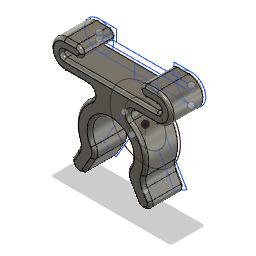
rPi Cable Clip IKEA JANSJO (Autodesk Fusion 360 design; units mm, degrees)
Autodesk Fusion 360 part; units mm, degrees
note: some values were not read from the file. Chosen so that the rebuilt part matches the saved one: a direction. Set by a fixed rule: which sketch regions a step uses.
sketch "Sketch1" plane through (0, 0, 0) normal (0, 0, 1) x (1, 0, 0) in component "Clip"
  circle A0 centre (0, 0) radius 3.6
  circle A1 centre (0, 0) radius 6.1
  line L0 (-1.8246, 8.2256) -> (2.1754, 8.2256)
  line L1 (2.1754, 8.2256) -> (2.1754, 5.6989)
  line L2 (2.1754, 5.6989) -> (-1.8246, 5.6989)
  line L3 (-1.8246, 5.6989) -> (-1.8246, 8.2256)
  line L4 (-8, 9.8345) -> (8, 9.8345)
  line L5 (8, 9.8345) -> (8, 8.8345)
  line L6 (8, 8.8345) -> (-8, 8.8345)
  line L7 (-8, 8.8345) -> (-8, 9.8345)
  circle A2 centre (-8, 9.3345) radius 0.5
  circle A3 centre (8, 9.3345) radius 0.5
  circle A4 centre (-8, 9.3345) radius 2.5
  circle A5 centre (8, 9.3345) radius 2.5
  line L8 (-8, 11.8345) -> (-5, 11.8345)
  line L9 (-5, 11.8345) -> (-5, 9.8345)
  line L10 (-5, 9.8345) -> (-8, 9.8345)
  line L11 (8, 11.8345) -> (5, 11.8345)
  line L12 (5, 11.8345) -> (5, 9.8345)
  line L13 (5, 9.8345) -> (8, 9.8345)
  line L14 (-8, 6.8345) -> (8, 6.8345)
  line L15 (8, 8.8345) -> (-8, 8.8345)
  line L16 (2.3229, -2.7503) -> (5.0741, -7.4897)
  line L17 (5.0741, -7.4897) -> (7.2362, -6.2346)
  line L18 (7.2362, -6.2346) -> (3.5999, 0.0297)
  line L19 (0, 0) -> (0, -10) construction
  line L20 (-7.2362, -6.2346) -> (-3.5999, 0.0297)
  line L21 (-5.0741, -7.4897) -> (-7.2362, -6.2346)
  line L22 (-2.3229, -2.7503) -> (-5.0741, -7.4897)
  dimension "d1" = 7.2
  dimension "d2" = 12.2
  dimension "d3" = 4
  dimension "d4" = 2.5
  measures "d1" diameter of A0
  measures "d2" diameter of A1
extrude "Extrude1" add sketch "Sketch1" along normal blind 6 contours A0 A1 L16 L18 | A0 A1 L2 L3 L18 L20 | A0 A1 L20 L22 | A1 L16 L17 L18 | A1 L20 L21 L22 | A1 L1 L3 L14 | A1 L2 L3 | L0 L1 L3 L6 A4 A5 L14 L15 | L0 L1 L3 L14 | L4 L6 A2 A4 L10 L15 | L4 L6 A3 A5 L13 L15 | L4 A4 L8 L9 L10 | L4 A5 L11 L12 L13 picked at (-9.1496, 7.9129) picked at (9.8232, 9.1922) in component "Clip"
fillet "Fillet1" radius 1 4 edges at (5, 11.8345, 3) (5, 9.8345, 3) (-5, 11.8345, 3) (-5, 9.8345, 3) in component "Clip"
fillet "Fillet2" radius 1 4 edges at (7.2362, -6.2346, 3) (5.0741, -7.4897, 3) (-5.0741, -7.4897, 3) (-7.2362, -6.2346, 3) in component "Clip"
fillet "Fillet7" radius 1 4 edges at (2.1754, 5.6989, 3) (2.1754, 6.8345, 3) (-1.8246, 6.8345, 3) (-1.8246, 5.8207, 3) in component "Clip"
fillet "Fillet8" radius 2 2 edges at (-5.3345, -2.9586, 3) (5.3345, -2.9586, 3) in component "Clip"
fillet "Fillet9" radius 2 2 edges at (2.3229, -2.7503, 3) (-2.3229, -2.7503, 3) in component "Clip"
fillet "Fillet10" radius 0.5 34 edges at (0, 8.8345, 6) (-8.5, 9.3345, 6) (-7, 9.8345, 6) (-5.2929, 10.1274, 6) (-5.2929, 11.5416, 6) (-7, 11.8345, 6) (-10.5, 9.3345, 6) (-6.0229, 6.8345, 6) (-3.0914, 6.1331, 6) (-5.8228, 1.8179, 6) (-5.5898, -3.0144, 6) (-6.2936, -4.6109, 6) (-6.8358, -6.1283, 6) (-6.1551, -6.8621, 6) (-5.1803, -7.0893, 6) (-3.7989, -5.293, 6) (-2.7558, -2.9268, 6) (0, 3.6, 6) (2.7558, -2.9268, 6) (3.7989, -5.293, 6) (5.1803, -7.0893, 6) (6.1551, -6.8621, 6) (6.8358, -6.1283, 6) (6.2936, -4.6109, 6) (5.5898, -3.0144, 6) (5.8228, 1.8179, 6) (3.0914, 6.1331, 6) (6.0229, 6.8345, 6) (10.5, 9.3345, 6) (7, 11.8345, 6) (5.2929, 11.5416, 6) (5.2929, 10.1274, 6) (7, 9.8345, 6) (8.5, 9.3345, 6) in component "Clip"
fillet "Fillet11" radius 0.5 34 edges at (-6.2936, -4.6109, 0) (-6.8358, -6.1283, 0) (-6.1551, -6.8621, 0) (-5.1803, -7.0893, 0) (-3.7989, -5.293, 0) (-2.7558, -2.9268, 0) (0, 3.6, 0) (2.7558, -2.9268, 0) (3.7989, -5.293, 0) (5.1803, -7.0893, 0) (6.1551, -6.8621, 0) (6.8358, -6.1283, 0) (6.2936, -4.6109, 0) (5.5898, -3.0144, 0) (5.8228, 1.8179, 0) (3.0914, 6.1331, 0) (6.0229, 6.8345, 0) (10.5, 9.3345, 0) (7, 11.8345, 0) (5.2929, 11.5416, 0) (5.2929, 10.1274, 0) (7, 9.8345, 0) (8.5, 9.3345, 0) (0, 8.8345, 0) (-8.5, 9.3345, 0) (-7, 9.8345, 0) (-5.2929, 10.1274, 0) (-5.2929, 11.5416, 0) (-7, 11.8345, 0) (-10.5, 9.3345, 0) (-6.0229, 6.8345, 0) (-3.0914, 6.1331, 0) (-5.8228, 1.8179, 0) (-5.5898, -3.0144, 0) in component "Clip"
component "Clip" placed x (1, 0, 0) y (0, 1, 0) z (0, 0, 1) at (0, 0, 0)
